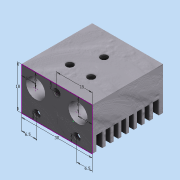
# Autodesk Inventor part: Chimera Heatsink
Saved by Autodesk Inventor 2016 (Build 200138000, 138)
## iProperties
Created: 2016-08-02
Part Number: Chimera Heatsink
Material: Aluminum 6061, Welded
Document SubType Name: Modeling
Designer: Sam
Density: 2.7 g/cm^3
Appearance: Weld - Aluminum
Author: Sam
Autodesk Inventor part; units mm, degrees
ref_plane "YZ Plane" through (0, 0, 0) normal (1, 0, 0) x (0, 1, 0)
ref_plane "XZ Plane" through (0, 0, 0) normal (0, 1, 0) x (-1, 0, 0)
ref_plane "XY Plane" through (0, 0, 0) normal (0, 0, 1) x (1, 0, 0)
sketch "Sketch2" plane through (0, 0, 0) normal (0, 1, 0) x (-1, 0, 0)
  line L0 (-8, 10) -> (22, 10)
  line L1 (22, 10) -> (22, -8)
  line L2 (22, -8) -> (-8, -8)
  line L3 (-8, -8) -> (-8, 10)
  point P0 (0, 0)
  point P1 (-2, 4)
  point P2 (16, 4)
  point P3 (7, 7)
  point P4 (15.5, -5)
  point P5 (-1.5, -5)
  dimension "d0" = 30
  dimension "d1" = 18
  dimension "d2" = 6
  dimension "d3" = 6
  dimension "d4" = 6
  dimension "d5" = 6
  dimension "d40" = 15
  dimension "d41" = 3
  dimension "d42" = 6.5
  dimension "d43" = 6.5
  dimension "d44" = 3
  dimension "d45" = 3
  constraints: 8 end point, 2 parallel, 1 horizontal, 1 perpendicular
  measures "d0" distance of L1.end L2.end
  measures "d1" distance of L0.end L1.end
  measures "d2" distance from line of L3 point (-2, 4)
  measures "d3" distance from line of L0 point (-2, 4)
  measures "d4" distance from line of L1 point (16, 4)
  measures "d5" distance from line of L0 point (16, 4)
  measures "d40" distance from line of L3 point (7, 7)
  measures "d41" distance from line of L0 point (7, 7)
  measures "d42" distance from line of point (-1.5, -5) L3
  measures "d43" distance from line of L1 point (15.5, -5)
  measures "d44" distance from line of point (-1.5, -5) L2
  measures "d45" distance from line of L2 point (15.5, -5)
extrude "Extrusion1" add sketch "Sketch2" along normal blind 30
hole "Hole1" at (2, 0, 4) at (-16, 0, 4) direction (0, 1, 0) diameter 7 end through all
hole "Hole2" at (-16, 0, 4) at (2, 0, 4) direction (0, 1, 0) diameter 8 depth 6.5 tip angle 118
sketch "Sketch3" plane through (8, 0, 10) normal (1, 0, 0) x (0, 0, -1)
  line L0 (18, 1.75) -> (12, 1.75)
  line L1 (12, 1.75) -> (12, 4.25)
  line L2 (12, 4.25) -> (18, 4.25)
  line L3 (18, 4.25) -> (18, 1.75)
  line L4 (18, 0) -> (0, 0) projected
  line L5 (18, 5.75) -> (12, 5.75)
  line L6 (12, 5.75) -> (12, 7.75)
  line L7 (12, 7.75) -> (18, 7.75)
  line L8 (18, 7.75) -> (18, 5.75)
  line L9 (18, 25.75) -> (12, 25.75)
  line L10 (12, 25.75) -> (12, 28.25)
  line L11 (12, 28.25) -> (18, 28.25)
  line L12 (18, 28.25) -> (18, 25.75)
  line L13 (18, 9.05) -> (12, 9.05)
  line L14 (12, 9.05) -> (12, 11.05)
  line L15 (12, 11.05) -> (18, 11.05)
  line L16 (18, 11.05) -> (18, 9.05)
  line L17 (18, 12.35) -> (12, 12.35)
  line L18 (12, 12.35) -> (12, 14.35)
  line L19 (12, 14.35) -> (18, 14.35)
  line L20 (18, 14.35) -> (18, 12.35)
  line L21 (18, 15.65) -> (12, 15.65)
  line L22 (12, 15.65) -> (12, 17.65)
  line L23 (12, 17.65) -> (18, 17.65)
  line L24 (18, 17.65) -> (18, 15.65)
  line L25 (18, 18.95) -> (12, 18.95)
  line L26 (12, 18.95) -> (12, 20.95)
  line L27 (12, 20.95) -> (18, 20.95)
  line L28 (18, 20.95) -> (18, 18.95)
  line L29 (18, 22.25) -> (12, 22.25)
  line L30 (12, 22.25) -> (12, 24.25)
  line L31 (12, 24.25) -> (18, 24.25)
  line L32 (18, 24.25) -> (18, 22.25)
  line L33 (0, 30) -> (18, 30) projected
  point P0 (10, 0)
  dimension "d22" = 6
  dimension "d23" = 2.5
  dimension "d24" = 1.75
  dimension "d25" = 6
  dimension "d26" = 2
  dimension "d27" = 1.5
  dimension "d36" = 6
  dimension "d37" = 2.5
  dimension "d46" = 6
  dimension "d47" = 2
  dimension "d48" = 1.3
  dimension "d49" = 6
  dimension "d50" = 2
  dimension "d51" = 6
  dimension "d52" = 2
  dimension "d53" = 6
  dimension "d54" = 2
  dimension "d55" = 6
  dimension "d56" = 2
  dimension "d57" = 1.75
  dimension "d58" = 1.5
  constraints: 64 end point, 16 parallel, 8 horizontal, 8 perpendicular
  measures "d22" distance of L1.end L2.end
  measures "d23" distance of L0.end L1.end
  measures "d24" distance between parallel lines of L0 L4
  measures "d25" distance of L6.end L7.end
  measures "d26" distance of L5.end L6.end
  measures "d27" distance between parallel lines of L2 L5
  measures "d36" distance of L10.end L11.end
  measures "d37" distance of L9.end L10.end
  measures "d46" distance of L14.end L15.end
  measures "d47" distance of L13.end L14.end
  measures "d48" distance between parallel lines of L7 L13
  measures "d49" distance of L18.end L20.start
  measures "d50" distance of L17.end L18.end
  measures "d51" distance of L22.end L24.start
  measures "d52" distance of L21.end L22.end
  measures "d53" distance of L26.end L28.start
  measures "d54" distance of L25.end L26.end
  measures "d55" distance of L30.end L32.start
  measures "d56" distance of L29.end L30.end
  measures "d57" distance between parallel lines of L33 L11
  measures "d58" distance between parallel lines of L31 L9
extrude "Extrusion3" cut sketch "Sketch3" against normal blind 30
hole "Hole3" at (-7, 0, 7) at (-15.5, 0, -5) at (1.5, 0, -5) direction (0, 1, 0) diameter 3 depth 10
thread "Thread1" size "M3x0.5" class "6H" standard "ANSI Metric M Profile" full length
thread "Thread2" size "M3x0.5" class "6H" standard "ANSI Metric M Profile" full length
thread "Thread3" size "M3x0.5" class "6H" standard "ANSI Metric M Profile" full length
sketch "Sketch4" plane through (-22, 0, 10) normal (0, 0, 1) x (1, 0, 0)
  line L0 (30, 0) -> (30, 30) projected
  line L1 (0, 30) -> (30, 30) projected
  point P0 (22, 0)
  point P1 (19.5, 10)
  point P2 (10.5, 10)
  point P3 (15, 20)
  dimension "d74" = 10.5
  dimension "d75" = 15
  dimension "d76" = 19.5
  dimension "d77" = 20
  dimension "d78" = 10
  measures "d74" distance from line of point (19.5, 10) L0
  measures "d75" distance from line of point (15, 20) L0
  measures "d76" distance from line of L0 point (10.5, 10)
  measures "d77" distance from line of L1 point (19.5, 10)
  measures "d78" distance from line of L1 point (15, 20)
hole "Hole4" at (-2.5, 10, 10) at (-11.5, 10, 10) at (-7, 20, 10) direction (0, 0, -1) diameter 3 depth 10
thread "Thread4" size "M3x0.5" class "6H" standard "ANSI Metric M Profile" full length
thread "Thread5" size "M3x0.5" class "6H" standard "ANSI Metric M Profile" full length
thread "Thread6" size "M3x0.5" class "6H" standard "ANSI Metric M Profile" full length
body "Solid1"
